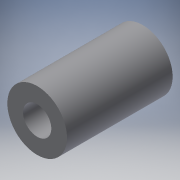
# Autodesk Inventor part: ditanciador 2.ipt-02
Saved by Autodesk Inventor 2018 (Build 220112000, 112)
## iProperties
Created: 2018-03-08
Part Number: ditanciador 2.ipt-02
Material: Generic
Document SubType Name: Modeling
Designer: isai
Density: 1 g/cm^3
Appearance: Default
Author: isai
Autodesk Inventor part; units mm, degrees
ref_plane "YZ Plane" through (0, 0, 0) normal (1, 0, 0) x (0, 1, 0)
ref_plane "XZ Plane" through (0, 0, 0) normal (0, 1, 0) x (-1, 0, 0)
ref_plane "XY Plane" through (0, 0, 0) normal (0, 0, 1) x (1, 0, 0)
sketch "Sketch1" plane through (0, 0, 0) normal (0, 0, 1) x (1, 0, 0)
  circle A0 centre (0, 33.9) radius 1.8 projected
  circle A1 centre (0, 33.9) radius 3.8
  point P0 (0, 0)
  dimension "d3" = 3.6
  constraints: 1 centre point
  measures "d3" diameter of A0
ref_plane "Work Plane1" through (-32, -22.1, 13.4512) normal (0, 0, -1) x (0, 1, 0)
extrude "Extrusion1" add sketch "Sketch1" along normal up to surface (13.4512 mm away)
equation "\"d\" = 4.2068"
body "Solid1"
